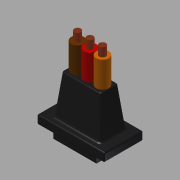
# Autodesk Inventor part: wire
Saved by Autodesk Inventor 2014 (Build 180170000, 170)
## iProperties
Created: 2013-07-13
Part Number: wire
Material: Generic
Document SubType Name: Modeling
Designer: Maurice
Density: 1 g/cm^3
Appearance: Default
Mass: 0.125693 g
Surface Area: 2.1283 cm^2
Volume: 0.125693 cm^3
Author: Maurice
Autodesk Inventor part; units mm, degrees
ref_plane "YZ Plane" through (0, 0, 0) normal (1, 0, 0) x (0, 1, 0)
ref_plane "XZ Plane" through (0, 0, 0) normal (0, 1, 0) x (-1, 0, 0)
ref_plane "XY Plane" through (0, 0, 0) normal (0, 0, 1) x (1, 0, 0)
sketch "Sketch1" plane through (0, 0, 0) normal (0, 1, 0) x (-1, 0, 0)
  line L0 (-2.5, -1.75) -> (2.5, -1.75)
  line L1 (2.5, -1.75) -> (2.5, 1.75)
  line L2 (2.5, 1.75) -> (-2.5, 1.75)
  line L3 (-2.5, 1.75) -> (-2.5, -1.75)
  line L4 (-2.5, -1.75) -> (2.5, 1.75) construction
  line L5 (2.5, -1.75) -> (-2.5, 1.75) construction
  point P0 (0, 0)
  dimension "d0" = 5
  dimension "d1" = 3.5
  constraints: 12 end point, 2 midpoint, 2 parallel, 1 horizontal, 1 perpendicular
  measures "d0" distance of L2.end L1.end
  measures "d1" distance of L1.end L0.end
extrude "Extrusion1" add sketch "Sketch1" along normal blind 1
sketch "Sketch2" plane through (0, 1, 0) normal (0, 1, 0) x (1, 0, 0)
  line L0 (-3.9, -2.25) -> (3.9, -2.25)
  line L1 (3.9, -2.25) -> (3.9, 2.25)
  line L2 (3.9, 2.25) -> (-3.9, 2.25)
  line L3 (-3.9, 2.25) -> (-3.9, -2.25)
  line L4 (-3.9, -2.25) -> (3.9, 2.25) construction
  line L5 (3.9, -2.25) -> (-3.9, 2.25) construction
  point P0 (0, 0)
  dimension "d4" = 7.8
  dimension "d5" = 4.5
  constraints: 12 end point, 2 midpoint, 2 parallel, 1 horizontal, 1 perpendicular
  measures "d4" distance of L2.end L1.end
  measures "d5" distance of L1.end L0.end
extrude "Extrusion2" add sketch "Sketch2" along normal blind 1
sketch "Sketch3" plane through (0, 2, 0) normal (0, 1, 0) x (1, 0, 0)
  line L0 (-2.75, -1.5) -> (2.75, -1.5)
  line L1 (2.75, -1.5) -> (2.75, 1.5)
  line L2 (2.75, 1.5) -> (-2.75, 1.5)
  line L3 (-2.75, 1.5) -> (-2.75, -1.5)
  line L4 (-2.75, -1.5) -> (2.75, 1.5) construction
  line L5 (2.75, -1.5) -> (-2.75, 1.5) construction
  point P0 (0, 0)
  dimension "d8" = 5.5
  dimension "d9" = 3
  constraints: 12 end point, 2 midpoint, 2 parallel, 1 horizontal, 1 perpendicular
  measures "d8" distance of L2.end L1.end
  measures "d9" distance of L1.end L0.end
extrude "Extrusion3" add sketch "Sketch3" along normal blind 4.5 draft -6
fillet "Fillet1" radius 0.3 8 edges at (2.5135, 4.25, 1.2635) (-2.5135, 4.25, 1.2635) (0, 2, 1.5) (2.75, 2, 0) (2.5135, 4.25, -1.2635) (0, 2, -1.5) (-2.5135, 4.25, -1.2635) (-2.75, 2, 0)
fillet "Fillet2" radius 0.15 20 edges at (0, 2, 2.25) (3.9, 2, 0) (0, 2, -2.25) (-3.9, 2, 0) (-3.9, 1, 0) (-3.9, 1.5, 2.25) (-3.9, 1.5, -2.25) (0, 1, -2.25) (3.9, 1.5, -2.25) (0, 1, 2.25) (3.9, 1.5, 2.25) (3.9, 1, 0) (-2.1898, 6.5, -0.9398) (-2.277, 6.5, 0) (-2.1898, 6.5, 0.9398) (0, 6.5, 1.027) (2.1898, 6.5, 0.9398) (2.277, 6.5, 0) (2.1898, 6.5, -0.9398) (0, 6.5, -1.027)
sketch "Sketch4" plane through (0, 6.5, 0) normal (0, 1, 0) x (1, 0, 0)
  circle A0 centre (0, 0) radius 0.72
  circle A1 centre (1.44, 0) radius 0.72
  circle A2 centre (-1.44, 0) radius 0.72
  dimension "d14" = 1.44
  dimension "d15" = 1.44
  dimension "d16" = 1.44
  constraints: 3 centre point, 2 equal radius, 2 horizontal alignment, 1 coincident
  measures "d14" diameter of A0
  measures "d15" diameter of A1
  measures "d16" diameter of A2
extrude "Extrusion4" add sketch "Sketch4" along normal blind 3
sketch "Sketch5" plane through (-1.44, 9.5, 0) normal (0, 1, 0) x (1, 0, 0)
  circle A0 centre (0, 0) radius 0.72 projected
  arc A1 (0.72, 0) -> (2.16, 0) centre (1.44, 0) ccw projected
  arc A2 (2.16, 0) -> (0.72, 0) centre (1.44, 0) ccw projected
  circle A3 centre (2.88, 0) radius 0.72 projected
  circle A4 centre (0, 0) radius 0.375
  circle A5 centre (1.44, 0) radius 0.375
  circle A6 centre (2.88, 0) radius 0.375
  dimension "d20" = 0.75
  dimension "d21" = 0.75
  constraints: 3 centre point, 3 coincident, 2 horizontal alignment, 1 equal radius
  measures "d20" diameter of A5
  measures "d21" diameter of A6
extrude "Extrusion5" add sketch "Sketch5" along normal blind 1 contours A4 | A5 | A6
body "Solid1"
